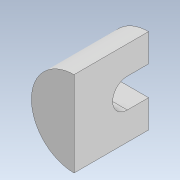
# Autodesk Inventor part: Gabel_Enforcement
Saved by Autodesk Inventor 2022 (Build 260153000, 153)
## iProperties
Created: 2022-10-11
Part Number: Gabel_Enforcement
Material: Generisch
Document SubType Name: Modeling
Designer: alexw
Density: 1 g/cm^3
Appearance: Vorgabe
Author: alexw
Autodesk Inventor part; units mm, degrees
ref_plane "YZ Plane" through (0, 0, 0) normal (1, 0, 0) x (0, 1, 0)
ref_plane "XZ Plane" through (0, 0, 0) normal (0, 1, 0) x (-1, 0, 0)
ref_plane "XY Plane" through (0, 0, 0) normal (0, 0, 1) x (1, 0, 0)
sketch "Skizze1" plane through (0, 0, 0) normal (0, 0, 1) x (1, 0, 0)
  circle A0 centre (0, 0) radius 8
  line L0 (0, -8) -> (0, 8)
  dimension "d0" = 16
  constraints: 2 end point, 2 point on circle, 1 centre point, 1 coincident, 1 midpoint, 1 vertical
  measures "d0" diameter of A0
extrude "Extrusion1" add sketch "Skizze1" along normal blind 14 contours L0 A0 picked at (-4.0721, -1.7428)
sketch "Skizze2" plane through (0, -8, 0) normal (1, 0, 0) x (0, 0, -1)
  line L0 (0, 0) -> (0, 16) construction
  line L1 (0, 16) -> (-14, 16) construction
  line L2 (-14, 0) -> (-14, 16) construction
  line L3 (0, 0) -> (-14, 0) construction
  line L4 (-14, 16) -> (-14, 0) construction
  line L5 (0, 16) -> (0, 0) construction
  line L6 (-14, 16) -> (0, 0) construction
  line L7 (0, 0) -> (-14, 0) construction
  line L8 (-14, 0) -> (0, 16) construction
  line L9 (-14, 8) -> (0, 8) construction
  point P0 (-4, 8)
  dimension "d12" = 4
  constraints: 6 end point, 1 midpoint, 1 perpendicular, 1 point on line
  measures "d12" distance from line of L0 point (-4, 8)
hole "Bohrung1" at (0, 0, 4) direction (-1, 0, 0) diameter 5.5 end through all clearance for "Inbusschraube DIN EN ISO 4762" size "M5" standard "DIN"
sketch "Skizze3" plane through (0, -8, 0) normal (1, 0, 0) x (0, 0, -1)
  circle A0 centre (-4, 8) radius 2.75
  line L0 (-4, 5.25) -> (0, 5.25)
  line L1 (0, 16) -> (0, 0) construction
  line L2 (-4, 10.75) -> (0, 10.75)
  line L3 (0, 5.25) -> (0, 10.75)
  circle A1 centre (-4, 8) radius 2.75 construction
  point P0 (0, 8)
  constraints: 6 end point, 3 tangent, 2 horizontal, 2 point on circle, 1 centre point, 1 concentric, 1 point on line, 1 vertical
extrude "Extrusion2" cut sketch "Skizze3" against normal through all contours A0 L2 L3 L0
